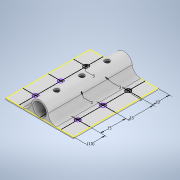
# Autodesk Inventor part: крепление направляющей руки
Saved by Autodesk Inventor 2020 (Build 240168000, 168)
## iProperties
Created: 2022-03-20
Part Number: крепление направляющей руки
Material: Типовые
Document SubType Name: Modeling
Designer: Администратор
Density: 1 g/cm^3
Appearance: По умолчанию
Author: Администратор
Autodesk Inventor part; units mm, degrees
ref_plane "YZ Plane" through (0, 0, 0) normal (1, 0, 0) x (0, 1, 0)
ref_plane "XZ Plane" through (0, 0, 0) normal (0, 1, 0) x (-1, 0, 0)
ref_plane "XY Plane" through (0, 0, 0) normal (0, 0, 1) x (1, 0, 0)
sketch "Эскиз1" plane through (0, 0, 0) normal (0, 0, 1) x (1, 0, 0)
  circle A0 centre (0, 0) radius 4
  circle A1 centre (0, 0) radius 5
  line L0 (-3, -4) -> (-20, -4)
  line L1 (-20, -4) -> (-20, -5)
  line L2 (-20, -5) -> (20, -5)
  line L3 (20, -5) -> (20, -4)
  line L4 (20, -4) -> (3, -4)
  line L5 (-5, 0) -> (-5, -4)
  line L6 (5, 0) -> (5, -4)
  dimension "d0" = 8
  dimension "d1" = 1
  dimension "d2" = 1
  dimension "d3" = 15
  dimension "d4" = 15
  constraints: 14 end point, 5 perpendicular, 4 point on circle, 4 point on line, 2 centre point, 2 tangent, 1 coincident, 1 horizontal
  measures "d0" diameter of A0
  measures "d1" radial gap between concentric circles of A0 A1
  measures "d2" distance of L0.end L1.end
  measures "d3" distance from line of L1.end L5
  measures "d4" distance from line of L3.end L6
extrude "Выдавливание1" add sketch "Эскиз1" along normal blind 50
sketch "Эскиз2" plane through (-20, -4, 0) normal (0, 1, 0) x (1, 0, 0)
  line L0 (15, 0) -> (0, 0) projected
  line L1 (15, 0) -> (0, 0) projected
  line L2 (0, 0) -> (0, -50) projected
  line L3 (15, -50) -> (0, -50) projected
  line L4 (15, 0) -> (15, -50) projected
  line L5 (40, 0) -> (25, 0) projected
  line L6 (25, 0) -> (25, -50) projected
  line L7 (40, -50) -> (25, -50) projected
  line L8 (40, 0) -> (40, -50) projected
  line L9 (25, 0) -> (15, 0) projected
  line L10 (15, 0) -> (15, -50) projected
  line L11 (25, -50) -> (15, -50) projected
  line L12 (25, 0) -> (25, -50) projected
  line L13 (40, 0) -> (25, 0) projected
  line L14 (32.5, 0) -> (32.5, -50)
  line L15 (40, -50) -> (25, -50) projected
  line L16 (7.5, 0) -> (7.5, -50)
  line L17 (15, -50) -> (0, -50) projected
  line L18 (20, 0) -> (20, -50)
  line L19 (15, -50) -> (25, -50) projected
  line L20 (40, -10) -> (0, -10)
  line L21 (0, 0) -> (0, -50) projected
  line L22 (0, -40) -> (40, -40)
  line L23 (40, 0) -> (40, -50) projected
  line L24 (40, -25) -> (0, -25)
  circle A0 centre (7.5, -10) radius 1.5
  circle A1 centre (20, -10) radius 1.5
  circle A2 centre (32.5, -10) radius 1.5
  circle A3 centre (32.5, -25) radius 1.5
  circle A4 centre (20, -25) radius 1.5
  circle A5 centre (7.5, -25) radius 1.5
  circle A6 centre (7.5, -40) radius 1.5
  circle A7 centre (20, -40) radius 1.5
  circle A8 centre (32.5, -40) radius 1.5
  dimension "d7" = 10
  dimension "d8" = 15
  dimension "d9" = 15
  dimension "d10" = 10
  dimension "d11" = 3
  dimension "d12" = 3
  dimension "d13" = 3
  dimension "d14" = 3
  constraints: 14 point on line, 12 end point, 12 midpoint, 9 centre point, 1 horizontal, 1 parallel
  measures "d7" distance between parallel lines of L20 L5
  measures "d8" distance between parallel lines of L24 L20
  measures "d9" distance between parallel lines of L22 L24
  measures "d10" distance between parallel lines of L7 L22
  measures "d11" diameter of A0
  measures "d12" diameter of A1
  measures "d13" diameter of A2
  measures "d14" diameter of A4
extrude "Выдавливание2" cut sketch "Эскиз2" against normal up to surface (1 mm away) contours A0 L20 L16 | L16 L20 A0 | A1 L18 L20 | L20 L18 A1 | A0 L16 L20 | A1 L20 L18 | L16 A0 L20 | A4 L18 L24 | L24 L18 A4 | A5 L16 L24 | L24 L16 A5 | L20 A1 L18 | A6 L16 L22 | L22 L16 A6 | A7 L18 L22 | L22 L18 A7 | L24 A4 L18 | L18 A4 L24 | L24 A5 L16 | L16 A5 L24 | A2 L20 L14 | L14 L20 A2 | L20 L14 A2 | L22 A6 L16 | L16 A6 L22 | L22 A7 L18 | L18 A7 L22 | L20 A2 L14 | A3 L14 L24 | L24 L14 A3 | A8 L14 L22 | L22 L14 A8 | L24 A3 L14 | L14 A3 L24 | L22 A8 L14 | L14 A8 L22
extrude "Выдавливание3" cut sketch "Эскиз2" along normal blind 50 contours A1 L18 L20 | L20 L18 A1 | A1 L20 L18 | A4 L18 L24 | L24 L18 A4 | L20 A1 L18 | A7 L18 L22 | L22 L18 A7 | L24 A4 L18 | L18 A4 L24 | L22 A7 L18 | L18 A7 L22
fillet "Сопряжение1" radius 5 2 edges at (5, -4, 25) (-5, -4, 25)
